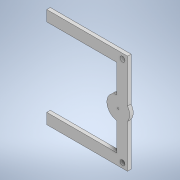
# Autodesk Inventor part: P7
Saved by Autodesk Inventor 2022 (Build 260153000, 153)
## iProperties
Created: 2022-11-21
Part Number: P7
Material: Genérico
Document SubType Name: Modeling
Designer: javie
Density: 1 g/cm^3
Appearance: Valor por defecto
Author: javie
Autodesk Inventor part; units mm, degrees
ref_plane "YZ Plane" through (0, 0, 0) normal (1, 0, 0) x (0, 1, 0)
ref_plane "XZ Plane" through (0, 0, 0) normal (0, 1, 0) x (-1, 0, 0)
ref_plane "XY Plane" through (0, 0, 0) normal (0, 0, 1) x (1, 0, 0)
sketch "Boceto1" plane through (0, 0, 0) normal (0, 0, 1) x (1, 0, 0)
  circle A0 centre (106.3631, -133) radius 3.5
  line L0 (0, -125) -> (98.3631, -125)
  line L1 (98.3631, -125) -> (98.3631, -85.8745)
  line L2 (0, -140) -> (0, -125)
  line L3 (0, 0) -> (113.3631, 0)
  line L4 (113.3631, 0) -> (113.3631, -60.6726)
  line L5 (0, -15) -> (0, 0)
  circle A1 centre (106.3631, -7) radius 3.5
  arc A2 (98.3631, -54.1255) -> (98.3631, -85.8745) centre (100.3631, -70) ccw
  line L6 (113.3631, -79.3274) -> (113.3631, -140)
  line L7 (113.3631, -140) -> (0, -140)
  line L8 (98.3631, -54.1255) -> (98.3631, -15)
  line L9 (98.3631, -15) -> (0, -15)
  arc A3 (113.3631, -79.3274) -> (113.3631, -60.6726) centre (100.3631, -70) ccw
  circle A4 centre (100.3631, -70) radius 1
  point P0 (98.3631, -85.8745)
  point P1 (113.3631, -79.3274)
  point P2 (113.3631, -60.6726)
  dimension "d0" = 2
  constraints: 20 end point, 5 centre point, 4 point on circle, 1 coincident
  measures "d0" diameter of A4
extrude "Extrusión1" add sketch "Boceto1" along normal blind 5
